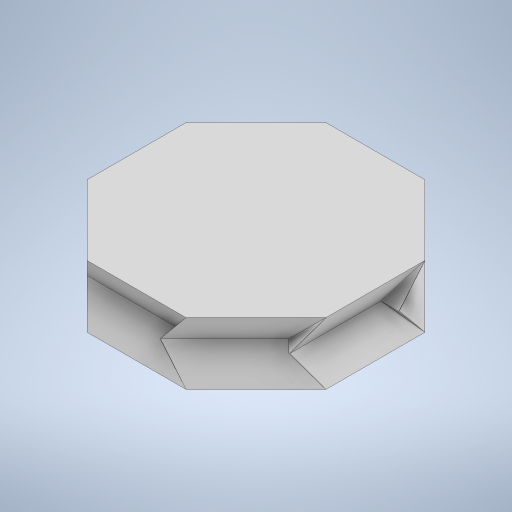
# Autodesk Inventor part: 팔각형 OV-PAM 층 한개
Saved by Autodesk Inventor 2024 (Build 280153000, 153)
## iProperties
Created: 2023-06-16
Part Number: 팔각형 OV-PAM 층 한개
Material: 일반
Document SubType Name: Modeling
Designer: jsw
Density: 1 g/cm^3
Appearance: 기본값
Mass: 146.501 g
Surface Area: 230.919 cm^2
Volume: 146.501 cm^3
Author: jsw
Autodesk Inventor part; units mm, degrees
ref_plane "YZ Plane" through (0, 0, 0) normal (1, 0, 0) x (0, 1, 0)
ref_plane "XZ Plane" through (0, 0, 0) normal (0, 1, 0) x (-1, 0, 0)
sketch "스케치1" plane through (0, 0, 0) normal (0, 1, 0) x (-1, 0, 0)
  line L0 (-45.4922, 18.8435) -> (-18.8435, 45.4922)
  line L1 (-18.8435, 45.4922) -> (18.8435, 45.4922)
  line L2 (18.8435, 45.4922) -> (45.4922, 18.8435)
  line L3 (45.4922, 18.8435) -> (45.4922, -18.8435)
  line L4 (45.4922, -18.8435) -> (18.8435, -45.4922)
  line L5 (18.8435, -45.4922) -> (-18.8435, -45.4922)
  line L6 (-18.8435, -45.4922) -> (-45.4922, -18.8435)
  line L7 (-45.4922, -18.8435) -> (-45.4922, 18.8435)
  line L8 (-19.092, 46.0922) -> (19.092, 46.0922)
  line L9 (19.092, 46.0922) -> (46.0922, 19.092)
  line L10 (46.0922, 19.092) -> (46.0922, -19.092)
  line L11 (46.0922, -19.092) -> (19.092, -46.0922)
  line L12 (19.092, -46.0922) -> (-19.092, -46.0922)
  line L13 (-19.092, -46.0922) -> (-46.0922, -19.092)
  line L14 (-46.0922, -19.092) -> (-46.0922, 19.092)
  line L15 (-46.0922, 19.092) -> (-19.092, 46.0922)
  point P0 (0, 0)
  point P1 (0, 0)
  point P2 (0, 0)
  dimension "d2" = 0.6
  dimension "d53" = 38.184
  constraints: 32 end point, 2 coincident, 2 horizontal, 34 other
  measures "d2" distance between parallel lines of L10 L3
  measures "d53" distance of L8.start L8.end
extrude "돌출2" add sketch "스케치1" along normal blind 12 contours L0 L1 L2 L3 L4 L5 L6 L7 | L8 L9 L10 L11 L12 L13 L14 L15
ref_plane "작업 평면2" through (46.0922, 0, 19.092) normal (-0.8660254, -0.5, 0) x (0, 0, -1)
sketch "스케치3" plane through (46.0922, 0, 19.092) normal (1, 0, 0) x (0, 0, -1)
  line L0 (0, 0) -> (0, 12) projected
  line L1 (0, 12) -> (38.184, 12) projected
  line L2 (0, 0) -> (38.184, 0)
  line L3 (38.184, 0) -> (38.184, 12)
  line L4 (38.184, 12) -> (0, 12)
  line L5 (0, 12) -> (0, 0)
  line L6 (0, 12) -> (-7.3047, 12)
  line L7 (-27.0002, 12) -> (0, 12) projected
  line L8 (0, 0) -> (-7.3047, 12)
  line L9 (38.184, 12) -> (19.092, 12)
  line L10 (28.092, 12) -> (38.184, 0)
  point P0 (19.092, 0)
  dimension "d17" = 121.33
  dimension "d49" = 9
  constraints: 16 end point, 5 midpoint, 2 parallel, 2 point on line, 1 horizontal, 1 perpendicular
  measures "d17" angle of L8 L2
  measures "d49" distance of point (19.092, 12) L10.start
extrude "돌출4" cut sketch "스케치3" along normal up to surface contours L8 L6 L0 | L0 L1 L10 L2 surface through (46.0922, 0, 19.092) normal (-0.8660254, -0.5, 0)
pattern_circular "원형 패턴1" count 8 over 360 about axis through (0, -10, 0) along (0, 1, 0) of "돌출4"
mirror "미러5" about plane through (0, 12, 0) normal (0, 1, 0) of "돌출2", "돌출4", "원형 패턴1"
